DHEClockingbottom (Autodesk Fusion 360 design; units mm, degrees)
Autodesk Fusion 360 part; units mm, degrees
sketch "Sketch1" plane through (0, 0, 0) normal (0, 0, 1) x (1, 0, 0)
  circle A0 centre (0, 0) radius 45
  circle A1 centre (0, 0) radius 47
  circle A2 centre (0, 0) radius 38.5
  dimension "d1" = 77
  dimension "d2" = 90
  dimension "d3" = 2
  constraint coincident A0.centre A1.centre
  constraint concentric A0 A1
  constraint concentric A1 A2
  measures "d1" diameter of A2
  measures "d2" diameter of A0
  measures "d3" distance of A0 A1
extrude "Extrude1" add sketch "Sketch1" along normal blind 10 contours A1
extrude "Extrude2" add sketch "Sketch1" against normal blind 5 contours A0 | A1
thread "Thread1" "BSP Pipe Threads G 2-11" major diameter 59.614 minor diameter 56.976 pitch 2.3091 angle 55 resizes the face on face at (38.3087, -3.8334, -1.6667)
sketch "Sketch2" plane through (0, 0, -5) normal (0, 0, -1) x (1, 0, 0)
  circle A0 centre (0, 0) radius 28.488
  circle A1 centre (0, 0) radius 47
  line L0 (30, 7.5) -> (35, 7.5)
  line L1 (35, 7.5) -> (35, -7.5)
  line L2 (35, -7.5) -> (30, -7.5)
  line L3 (30, -7.5) -> (30, 7.5)
  line L4 (-46.3977, -7.5) -> (-46.3977, 7.5)
  line L5 (-41.3977, 7.5) -> (-41.3977, -7.5)
  line L6 (-41.3977, -7.5) -> (-46.3977, -7.5)
  line L7 (-46.3977, 7.5) -> (-41.3977, 7.5)
  point P0 (30, 0)
  dimension "d8" = 5
  dimension "d9" = 15
  dimension "d10" = 30
  dimension "d15" = 5
  dimension "d16" = 15
  constraint horizontal L0
  constraint vertical L1
  constraint horizontal L2
  constraint vertical L3
  constraint midpoint L3 P0
  constraint horizontal A0.centre P0
  constraint coincident A1 L4.start
  constraint coincident A1 L4.end
  constraint vertical L4
  constraint parallel L4 L5
  constraint perpendicular L4 L6
  constraint perpendicular L5 L7
  measures "d8" distance of L1 L3
  measures "d9" distance of L0 L2
  measures "d10" distance of A0.centre L3
  measures "d15" distance of L4 L5
  measures "d16" distance of L6 L7
extrude "Extrude3" add sketch "Sketch2" along normal blind 15 contours L4 L5 L6 L7 | L0 L1 L2 L3
sketch "Sketch3" plane through (35, 0, 0) normal (1, 0, 0) x (0, 1, 0)
  line L0 (7.5, -5) -> (-7.5, -5)
  line L1 (-7.5, -5) -> (-7.5, -20)
  line L2 (-7.5, -20) -> (7.5, -20)
  line L3 (7.5, -20) -> (7.5, -5)
  circle A0 centre (0, -12.5) radius 7.5
  circle A1 centre (0, -12.5) radius 5
  dimension "d13" = 10
  constraint tangent L2 A0
  constraint concentric A0 A1
  constraint tangent L1 A0
  constraint tangent L3 A0
  measures "d13" diameter of A1
extrude "Extrude4" cut sketch "Sketch3" against normal through all contours L2 L3 A0 | L1 L2 A0 | A1
